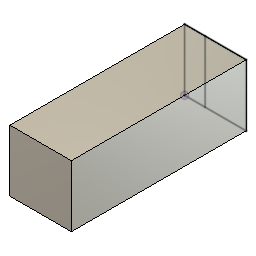
Hook+Holder (Autodesk Fusion 360 design; units mm, degrees)
Autodesk Fusion 360 part; units mm, degrees
sketch "Sketch1" plane through (0, 0, 0) normal (0, 0, 1) x (1, 0, 0)
  line L0 (0, 0) -> (22.352, 0)
  line L1 (22.352, 0) -> (22.352, 22.352)
  line L2 (22.352, 22.352) -> (0, 22.352)
  line L3 (0, 22.352) -> (0, 0)
  line L4 (7.4507, 22.352) -> (7.4507, 0)
  dimension "d1" = 22.352
  dimension "d2" = 22.352
  dimension "d3" = 7.4507
  constraint horizontal L0
  constraint vertical L1
  constraint horizontal L2
  constraint vertical L3
  constraint coincident L0.start L3.end
  constraint coincident L2 L4.start
  constraint coincident L0 L4.end
  constraint perpendicular L0 L4
  measures "d1" distance of L0.start L0.end
  measures "d2" distance of L0.start L2.end
  measures "d3" distance of L3 L4
extrude "Extrude1" add sketch "Sketch1" along normal blind 63.5 contours L0 L2 L3 L4
sketch "Sketch2" plane through (7.4507, 0, 0) normal (1, 0, 0) x (0, 0, -1)
  line L0 (0, 0) -> (0, 22.352)
  line L1 (0, 22.352) -> (-63.5, 22.352)
  line L2 (-63.5, 22.352) -> (-63.5, 0)
  line L3 (-63.5, 0) -> (0, 0)
  line L4 (-50.8, 0) -> (-50.8, 19.1554)
  line L5 (-50.8, 19.1554) -> (-17.6219, 0)
  dimension "d6" = 12.7
  dimension "d7" = 30
  constraint coincident L3 L4.start
  constraint perpendicular L3 L4
  constraint coincident L3 L5.end
  measures "d6" distance of L2 L4
  measures "d7" angle of L3 L5
extrude "Extrude2" add sketch "Sketch2" along normal blind 7.4507 contours L0 L1 L2 L3 L4 L5
sketch "Sketch3" plane through (14.9013, 0, 0) normal (1, 0, 0) x (0, 0, -1)
  line L0 (-50.8, 19.1554) -> (-17.6219, 0)
  line L1 (-17.6219, 0) -> (0, 0)
  line L2 (0, 0) -> (0, 22.352)
  line L3 (0, 22.352) -> (-63.5, 22.352)
  line L4 (-63.5, 22.352) -> (-63.5, 0)
  line L5 (-63.5, 0) -> (-50.8, 0)
  line L6 (-50.8, 0) -> (-50.8, 19.1554)
  line L7 (-63.5, 0) -> (0, 0)
  line L8 (0, 0) -> (0, 22.352)
  line L9 (0, 22.352) -> (-63.5, 22.352)
  line L10 (-63.5, 22.352) -> (-63.5, 0)
  constraint horizontal L7
  constraint vertical L8
  constraint horizontal L9
  constraint vertical L10
  constraint coincident L2.end L3.start
  constraint coincident L4.end L5.start
extrude "Extrude3" add sketch "Sketch3" along normal blind 7.4507
equation "d3 = ( 0.88 / 3 ) * 1 in"
equation "d8 = ( 0.88 / 3 ) * 1 in"
equation "d10 = ( 0.88 / 3 ) * 1 in"
